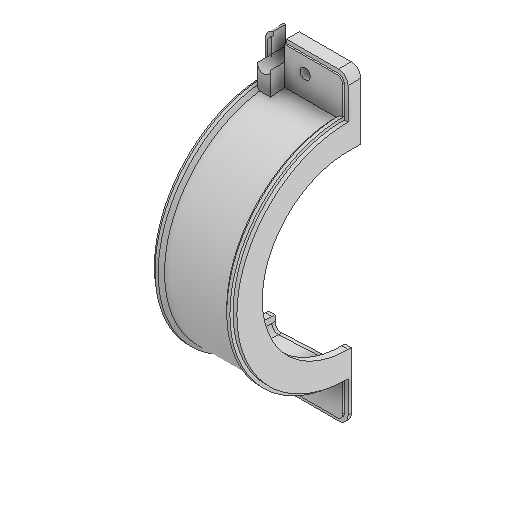
# Autodesk Inventor part: Test
Saved by Autodesk Inventor 2025.3 (Build 293356030, 356C)
## iProperties
Created: 2025-04-17
Part Number: Test
Material: Generic
Document SubType Name: Modeling
Designer: Andreas
Density: 1 g/cm^3
Appearance: Default
Author: Andreas
Autodesk Inventor part; units mm, degrees
ref_plane "YZ Plane" through (0, 0, 0) normal (1, 0, 0) x (0, 1, 0)
ref_plane "XZ Plane" through (0, 0, 0) normal (0, 1, 0) x (-1, 0, 0)
sketch "Sketch1" plane through (0, 0, 0) normal (0, 0, 1) x (1, 0, 0)
  line L0 (0, 30) -> (0, 31.907)
  line L1 (2.0908, 33.905) -> (18, 33.1818)
  line L2 (22, 29.5) -> (22, 27)
  line L3 (22, 27) -> (24, 27)
  line L4 (24, 27) -> (24, 35)
  line L5 (-2, 35) -> (-2, 30)
  line L6 (-2, 30) -> (0, 30)
  line L7 (0, 0) -> (88.4682, 0)
  arc A0 (2.0908, 33.905) -> (0, 31.907) centre (2, 31.907) ccw
  line L8 (18, 33.1818) -> (22, 29.5)
  line L9 (-2, 35) -> (-0.8, 35)
  line L10 (-0.8, 35) -> (-0.8, 36)
  line L11 (-0.8, 36) -> (0.2, 36)
  line L12 (0.2, 36) -> (0.2, 35)
  line L13 (0.2, 35) -> (21.8, 35)
  line L14 (21.8, 35) -> (21.8, 36)
  line L15 (24, 35) -> (22.8, 35)
  line L16 (22.8, 35) -> (22.8, 36)
  line L17 (22.8, 36) -> (21.8, 36)
  point P0 (0, 34)
  point P1 (22, 33)
  point P2 (-1, 30)
  point P3 (22.3, 36)
  point P4 (-0.3, 36)
  dimension "d0" = 66
  dimension "d1" = 68
  dimension "d2" = 22
  dimension "d3" = 2
  dimension "d4" = 6
  dimension "d7" = 2
  dimension "d8" = 4
  dimension "d9" = 3.5
  dimension "d10" = 4
  dimension "d11" = 2
  dimension "d12" = 1.2
  dimension "d13" = 70
  dimension "d14" = 1
  dimension "d16" = 26
  dimension "d66" = 1
  constraints: 36 end point, 8 perpendicular, 4 equal length, 4 horizontal, 4 point on line, 3 midpoint, 3 vertical, 2 point on circle, 2 tangent, 1 centre point, 1 horizontal alignment, 1 parallel, 1 vertical alignment
  measures "d0" diameter of point (22, 33) L7
  measures "d1" diameter of point (0, 34) L7
  measures "d2" horizontal distance of point (0, 34) point (22, 33)
  measures "d3" distance of L2.end L3.end
  measures "d4" distance from line of point (22, 33) L3
  measures "d7" radius of A0
  measures "d8" horizontal distance of L1.end point (22, 33)
  measures "d9" distance of L2.start point (22, 33)
  measures "d10" vertical distance of point (0, 34) point (-1, 30)
  measures "d11" distance of L5.end L0.start
  measures "d12" distance of L5.start L9.end
  measures "d13" diameter of L9 L7
  measures "d14" distance of L11.end L12.end
  measures "d16" distance between parallel lines of L4 L5
  measures "d66" distance of L10.end L11.end
revolve "Revolution1" add sketch "Sketch1" angle 180 about axis through (0, 0, 0) along (1, 0, 0)
sketch "Sketch2" plane through (21.8, -35, 0) normal (0, 0, -1) x (-1, 0, 0)
  line L0 (23.8, 0) -> (23.8, 5) projected
  line L1 (23.8, 0) -> (-2.2, 0)
  line L2 (-2.2, 0) -> (-2.2, -10)
  line L3 (0.8, -13) -> (20.8, -13)
  line L4 (23.8, -10) -> (23.8, 0)
  arc A0 (20.8, -13) -> (23.8, -10) centre (20.8, -10) ccw
  arc A1 (-2.2, -10) -> (0.8, -13) centre (0.8, -10) ccw
  line L5 (23.8, 5) -> (21.8, 5) projected
  line L6 (21.8, 5) -> (21.8, 3.093) projected
  arc A2 (19.7092, 1.095) -> (21.8, 3.093) centre (19.8, 3.093) ccw projected
  line L7 (19.7092, 1.095) -> (3.8, 1.8182) projected
  line L8 (3.8, 1.8182) -> (-0.2, 5.5) projected
  line L9 (-0.2, 5.5) -> (-0.2, 8) projected
  line L10 (-0.2, 8) -> (-2.2, 8) projected
  line L11 (-2.2, 8) -> (-2.2, 0) projected
  line L12 (-2.2, 0) -> (-1, 0) projected
  line L13 (-1, 0) -> (-1, -1) projected
  line L14 (-1, -1) -> (0, -1) projected
  line L15 (0, -1) -> (0, 0) projected
  line L16 (0, 0) -> (21.6, 0) projected
  line L17 (21.6, 0) -> (21.6, -1) projected
  line L18 (21.6, -1) -> (22.6, -1) projected
  line L19 (22.6, -1) -> (22.6, 0) projected
  line L20 (22.6, 0) -> (23.8, 0) projected
  line L21 (23.8, 0) -> (23.8, 5) projected
  point P0 (21.8, 35)
  dimension "d17" = 48
  dimension "d18" = 3
  constraints: 8 end point, 4 point on circle, 4 tangent, 2 centre point, 2 parallel, 1 coincident, 1 equal radius, 1 horizontal, 1 perpendicular
  measures "d17" distance from line of point (21.8, 35) L3
  measures "d18" radius of A0
extrude "Extrusion1" add sketch "Sketch2" along normal blind 1
sketch "Sketch3" plane through (21.8, -35, 0) normal (0, 0, 1) x (1, 0, 0)
  line L0 (-23.8, -10) -> (-23.8, 0) projected
  arc A0 (-23.8, -10) -> (-20.8, -13) centre (-20.8, -10) ccw projected
  line L1 (-0.8, -13) -> (-20.8, -13) projected
  arc A1 (-0.8, -13) -> (2.2, -10) centre (-0.8, -10) ccw projected
  line L2 (2.2, 0) -> (2.2, -10) projected
  line L3 (0, 0) -> (-21.6, 0) projected
  line L4 (0, -1) -> (0, 71) projected
  line L5 (-21.6, -1) -> (-21.6, 71) projected
  line L6 (-22.6, 0) -> (-22.6, -10)
  arc A2 (-22.6, -10) -> (-20.8, -11.8) centre (-20.8, -10) ccw
  line L7 (-20.8, -11.8) -> (-0.8, -11.8)
  arc A3 (-0.8, -11.8) -> (1, -10) centre (-0.8, -10) ccw
  line L8 (1, -10) -> (1, 0)
  line L9 (-21.6, -1) -> (-22.6, -1) projected
  line L10 (1, -1) -> (0, -1) projected
  point P0 (-21.8, 35)
  point P1 (-21.6, 71)
  constraints: 6 end point, 4 point on circle, 2 centre point, 1 point on line, 5 other
extrude "Extrusion2" add sketch "Sketch3" along normal blind 0.5
sketch "Sketch4" plane through (21.8, -35, -1) normal (0, 0, -1) x (-1, 0, 0)
  line L0 (0.8, -13) -> (20.8, -13) projected
  point P0 (21.8, 35)
  point P1 (10.8, -7)
  point P2 (10.8, -13)
  dimension "d30" = 42
  constraints: 1 midpoint, 1 vertical alignment
  measures "d30" vertical distance of point (21.8, 35) point (10.8, -7)
hole "Hole1" at (11, -42, -1) direction (0, 0, 1) diameter 3.2 depth 4.5 tip angle 118
mirror "Mirror1" about plane through (0, 0, 0) normal (0, 1, 0) of "Extrusion1", "Extrusion2", "Hole1"
sketch "Sketch5" plane through (21, 48, -1) normal (0, 0, -1) x (-1, 0, 0)
  line L0 (23, -3) -> (23, -18) projected
  line L1 (0, 0) -> (20, 0) projected
  point P0 (21, -48)
  point P1 (18.5, -6)
  dimension "d38" = 4.5
  dimension "d39" = 6
  measures "d38" distance from line of L0 point (18.5, -6)
  measures "d39" distance from line of L1 point (18.5, -6)
hole "Hole2" at (2.5, 42, -1) direction (0, 0, 1) diameter 4.2 depth 8 tip angle 118
chamfer "Chamfer1" distance 1 angle 45 2 edges at (21.8, 0, 35) (0.2, 0, 35)
sketch "Sketch6" plane through (0.2, 35, 0.5) normal (0, 0, 1) x (1, 0, 0)
  circle A0 centre (2.3, 7) radius 2.1 projected
  line L0 (4.4, 7) -> (0.2, 7)
  line L1 (0.2, 7) -> (0.2, -1.0182)
  line L2 (0.2, -1.0182) -> (4.4, -1.2091)
  line L3 (4.4, -1.2091) -> (4.4, 7)
  line L4 (21.6, 0) -> (0, 0) projected
  line L5 (1.8908, -1.095) -> (17.8, -1.8182) projected
  point P0 (-0.2, -35)
  point P1 (0.2, 7)
  point P2 (4.1466, 0)
  point P3 (0.4534, 0)
  constraints: 8 end point, 2 point on line, 2 vertical, 1 horizontal, 1 parallel, 1 perpendicular, 2 other
extrude "Extrusion3" add sketch "Sketch6" along normal blind 4.5 contours L3 L4 L1 A0 | L3 L2 L1 L4
sketch "Sketch7" plane through (1, 46.8, 0.5) normal (0, 0, 1) x (1, 0, 0)
  line L0 (3.6, -12.159) -> (3.6, -4.8) projected
  line L1 (3.6, -4.8) -> (-0.6, -4.8)
  line L2 (-0.6, -4.8) -> (-0.6, 4.5267)
  line L3 (-0.6, 4.5267) -> (3.6, 4.5267)
  line L4 (3.6, 4.5267) -> (3.6, -4.8)
  point P0 (-1, -46.8)
  constraints: 8 end point, 2 parallel, 1 horizontal, 1 perpendicular
extrude "Extrusion4" cut sketch "Sketch7" against normal blind 4.5
ref_plane "Work Plane1" through (-0.8, 0, 36) normal (0, 0, 1) x (1, 0, 0)
sketch "Sketch8" plane through (-0.8, 0, 36) normal (0, 0, 1) x (1, 0, 0)
  line L0 (0.8, -30) -> (0.8, 30) projected
  line L1 (22.6, -35.9965) -> (22.6, 35.9965) projected
  line L2 (0.8, 2) -> (22.6, 2)
  line L3 (22.6, 2) -> (22.6, -2)
  line L4 (22.6, -2) -> (0.8, -2)
  line L5 (0.8, -2) -> (0.8, 2)
  circle A0 centre (11.7, 0) radius 3
  line L6 (1, -35.9965) -> (1, 35.9965) projected
  point P0 (0.8, 0)
  point P1 (0.8, 0)
  point P2 (11.7, -2)
  point P3 (1, 0)
  point P4 (1, 35.9965)
  point P5 (1, -35.9965)
  point P6 (13.9361, -2)
  point P7 (13.9361, 2)
  point P8 (9.4639, 2)
  point P9 (0.8, -2)
  point P10 (9.4639, -2)
  dimension "d47" = 4
  dimension "d48" = 6
  constraints: 8 end point, 3 midpoint, 2 parallel, 2 point on line, 1 centre point, 1 horizontal, 1 horizontal alignment, 1 perpendicular, 1 vertical alignment, 2 other
  measures "d47" distance between parallel lines of L2 L4
  measures "d48" diameter of A0
extrude "Extrusion5" [suppressed]
sketch "Sketch9" plane through (-0.8, 0, 36) normal (0, 0, 1) x (1, 0, 0)
  line L0 (22.6, -2) -> (22.6, 0) projected
  line L1 (22.6, 0) -> (22.6, 2) projected
  line L2 (22.6, 2) -> (13.9361, 2) projected
  arc A0 (13.9361, 2) -> (9.4639, 2) centre (11.7, 0) ccw projected
  line L3 (9.4639, 2) -> (0.8, 2) projected
  line L4 (0.8, 2) -> (0.8, 0) projected
  line L5 (0.8, 0) -> (0.8, -2) projected
  line L6 (0.8, -2) -> (9.4639, -2) projected
  arc A1 (9.4639, -2) -> (13.9361, -2) centre (11.7, 0) ccw projected
  line L7 (13.9361, -2) -> (22.6, -2) projected
  line L8 (0.8, 1) -> (22.6, 1)
  line L9 (22.6, 1) -> (22.6, -1)
  line L10 (22.6, -1) -> (0.8, -1)
  line L11 (0.8, -1) -> (0.8, 1)
  circle A2 centre (11.7, 0) radius 3
  point P0 (0.8, 0)
  point P1 (14.5284, 1)
  point P2 (14.5284, -1)
  point P3 (8.8716, 1)
  point P4 (9.4639, 2)
  point P5 (9.4639, -2)
  point P6 (8.8716, -1)
  point P7 (0.8, -1)
  constraints: 8 end point, 2 midpoint, 2 parallel, 1 coincident, 1 horizontal, 1 perpendicular, 3 other
extrude "Extrusion6" [suppressed]
chamfer "Chamfer2" [suppressed]
sketch "Sketch10" plane through (-0.8, 0, 36) normal (0, 0, 1) x (1, 0, 0)
  arc A0 (13.9361, 2) -> (9.4639, 2) centre (11.7, 0) ccw projected
  point P0 (0.8, 0)
  constraints: 1 coincident
hole "Hole3" [suppressed]
chamfer "Chamfer3" [suppressed]
sketch "Sketch11" plane through (24, 27, -1) normal (0, 0, -1) x (-1, 0, 0)
  line L0 (23.6, 20.9394) -> (23.6, 15) projected
  arc A0 (19.4, 15) -> (23.6, 15) centre (21.5, 15) ccw projected
  line L1 (19.4, 15) -> (19.4, 21) projected
  line L2 (3, 21) -> (19.4, 21) projected
  arc A1 (3, 21) -> (0, 18) centre (3, 18) ccw projected
  line L3 (0, 0) -> (0, 18) projected
  line L4 (2, 0) -> (0, 0) projected
  line L5 (2, 2.5) -> (2, 0) projected
  line L6 (6, 6.1818) -> (2, 2.5) projected
  line L7 (21.9092, 6.905) -> (6, 6.1818) projected
  arc A2 (24, 4.907) -> (21.9092, 6.905) centre (22, 4.907) ccw projected
  line L8 (24, 3) -> (24, 4.907) projected
  line L9 (26, 3) -> (24, 3) projected
  line L10 (26, 18) -> (26, 3) projected
  arc A3 (26, 18) -> (23.6, 20.9394) centre (23, 18) ccw projected
  circle A4 centre (13, 15) radius 1.6 projected
  point P0 (24, -27)
extrude "Extrusion7" add sketch "Sketch11" along normal blind 3
equation "\"d17\" = 0.5 * Outer_Diameter"
equation "\"Outer_Diameter\" = 96"
body "Solid1"
